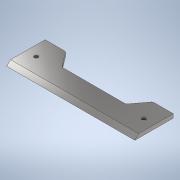
# Autodesk Inventor part: HM_Knife_cut
Saved by Autodesk Inventor 2021 (Build 250183000, 183)
## iProperties
Created: 2020-12-06
Part Number: HM_Knife_cut
Material: Steel, Alloy
Document SubType Name: Modeling
Designer: ermoz
Density: 7.73 g/cm^3
Appearance: Semi-Polished
Author: ermoz
Autodesk Inventor part; units mm, degrees
ref_plane "YZ Plane" through (0, 0, 0) normal (1, 0, 0) x (0, 1, 0)
ref_plane "XZ Plane" through (0, 0, 0) normal (0, 1, 0) x (-1, 0, 0)
ref_plane "XY Plane" through (0, 0, 0) normal (0, 0, 1) x (1, 0, 0)
sketch "Sketch1" plane through (0, 0, 0) normal (0, 1, 0) x (-1, 0, 0)
  line L0 (50, 15) -> (-50, 15)
  line L1 (-50, 15) -> (-50, -15)
  line L2 (-50, -15) -> (50, -15)
  line L3 (50, -15) -> (50, 15)
  line L4 (50, 15) -> (-50, -15) construction
  line L5 (-50, 15) -> (50, -15) construction
  point P0 (0, 0)
  dimension "d0" = 100
  dimension "d1" = 30
  constraints: 12 end point, 2 midpoint, 2 parallel, 1 horizontal, 1 perpendicular
  measures "d0" distance of L2.end L1.end
  measures "d1" distance of L1.end L0.end
extrude "Extrusion1" add sketch "Sketch1" along normal blind 3
sketch "Sketch2" plane through (50, 0, 15) normal (1, 0, 0) x (0, 0, -1)
  line L0 (0, 0) -> (3, 3)
  line L1 (0, 0) -> (4.2426, 0) construction
  line L2 (3, 3) -> (0, 3)
  line L3 (0, 0) -> (0, 3) projected
  line L4 (0, 3) -> (0, 0)
  dimension "d4" = 45
  constraints: 8 end point, 1 equal length, 1 horizontal, 1 perpendicular
  measures "d4" angle of L1 L0
extrude "Extrusion2" cut sketch "Sketch2" against normal blind 100
sketch "Sketch3" plane through (0, 0, 0) normal (0, -1, 0) x (1, 0, 0)
  line L0 (25, -15) -> (-25, -15)
  line L1 (-25, -15) -> (-25, -3)
  line L2 (-25, -3) -> (25, -3)
  line L3 (25, -3) -> (25, -15)
  line L4 (0, 0) -> (0, -9.0285)
  line L5 (50, -15) -> (-50, -15) projected
  circle A0 centre (42, 0) radius 1.5
  circle A1 centre (-42, 0) radius 1.5
  line L6 (25, -3) -> (34, -15)
  line L7 (34, -15) -> (25, -15)
  line L8 (-25, -3) -> (-34, -15)
  line L9 (-25, -15) -> (-34, -15)
  line L10 (50, 15) -> (50, -15) projected
  dimension "d7" = 50
  dimension "d8" = 12
  dimension "d9" = 0
  dimension "d10" = 3
  dimension "d12" = 15
  dimension "d19" = 9
  dimension "d20" = 9
  dimension "d21" = 8
  constraints: 18 end point, 2 centre point, 2 parallel, 2 point on line, 1 equal radius, 1 horizontal, 1 perpendicular, 1 symmetric about line, 1 vertical, 1 other
  measures "d7" distance of L0.start L0.end
  measures "d8" distance of L2.end L0.start
  measures "d9" distance between parallel lines of L5 L0
  measures "d10" diameter of A0
  measures "d12" distance from line of L5 A0.centre
  measures "d19" distance of L6.end L0.start
  measures "d20" distance of L0.end L8.end
  measures "d21" distance from line of L10 A0.centre
extrude "Extrusion3" cut sketch "Sketch3" against normal through all
chamfer "Chamfer1" distance 2 angle 45 2 edges at (40.5, 0, 0) (-43.5, 0, 0)
fillet "Fillet1" radius 2 4 edges at (-25, 1.5, -3) (25, 1.5, -3) (-34, 1.5, -15) (34, 1.5, -15)
body "Solid1"
